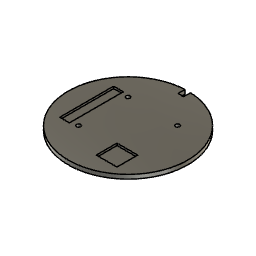
ASMBLY_NonSym v9 (Autodesk Fusion 360 archive; units mm, degrees)
design "Plate_Tag"
Autodesk Fusion 360 part; units mm, degrees
(part 1 of 2)
sketch "Sketch1" plane through (0, 0, 0) normal (0, 0, 1) x (1, 0, 0)
  circle A0 centre (0, 0) radius 43.3
  line L0 (17.936, 17.936) -> (-17.936, 17.936) construction
  line L1 (-17.936, 17.936) -> (-17.936, -17.936) construction
  line L2 (-17.936, -17.936) -> (17.936, -17.936) construction
  line L3 (17.936, -17.936) -> (17.936, 17.936) construction
  line L4 (17.936, 17.936) -> (-17.936, -17.936) construction
  line L5 (-17.936, 17.936) -> (17.936, -17.936) construction
  circle A1 centre (17.936, 17.936) radius 1.5
  line L6 (0, 17.936) -> (0, -17.936) construction
  line L7 (-17.936, 0) -> (17.936, 0) construction
  circle A2 centre (-17.936, 17.936) radius 1.5
  circle A3 centre (17.936, -17.936) radius 1.5
  circle A4 centre (-17.936, -17.936) radius 1.5
  line L8 (0, 43.3) -> (0, 38.2538) construction
  line L9 (0, 38.2538) -> (2, 38.2538)
  line L10 (2, 38.2538) -> (2, 43.2538)
  line L11 (-2, 38.2538) -> (-2, 43.2538)
  line L12 (0, 38.2538) -> (-2, 38.2538)
  line L13 (-23.936, 19.5) -> (-29.936, 19.5)
  line L14 (-29.936, 19.5) -> (-29.936, -19.5)
  line L15 (-29.936, -19.5) -> (-23.936, -19.5)
  line L16 (-23.936, -19.5) -> (-23.936, 19.5)
  line L17 (-23.936, 19.5) -> (-29.936, -19.5) construction
  line L18 (-29.936, 19.5) -> (-23.936, -19.5) construction
  point P0 (-26.936, 0)
  dimension "d1" = 86.6
  dimension "d2" = 35.872
  dimension "d3" = 35.872
  dimension "d4" = 3
  dimension "d7" = 4
  dimension "d8" = 5
  dimension "d9" = 6
  dimension "d10" = 39
  dimension "d26" = 12
  constraint coincident A0.centre origin
  constraint perpendicular L0 L1
  constraint parallel L0 L2
  constraint parallel L1 L3
  constraint horizontal L0
  constraint coincident L4 A0.centre
  constraint coincident L5 A0.centre
  constraint coincident L0.start L3.end
  constraint midpoint L0 L6.start
  constraint midpoint L2 L6.end
  constraint midpoint L1 L7.start
  constraint midpoint L3 L7.end
  constraint symmetric A1 L6 A2
  constraint symmetric A1 L7 A3
  constraint symmetric L7 A2 A4
  constraint coincident A0 L8.start
  constraint vertical L8
  constraint perpendicular L8 L9
  constraint coincident A0 L10.end
  constraint perpendicular L9 L10
  constraint collinear A0.centre L8.start L8.end
  constraint symmetric L9.start L8 L12.start
  constraint symmetric L8 L9.end L11.start
  constraint symmetric L8 L10.end L11.end
  constraint perpendicular L13 L14
  constraint parallel L13 L15
  constraint parallel L14 L16
  constraint horizontal L13
  constraint coincident L17 P0
  constraint coincident L18 P0
  constraint coincident L7 P0
  measures "d1" diameter of A0
  measures "d2" distance of L0.start L2.end
  measures "d3" distance of L0.start L0.end
  measures "d4" diameter of A1
  measures "d7" distance of L9.end L11.start
  measures "d8" distance of L9.end L10.end
  measures "d9" distance of L13.start L13.end
  measures "d10" distance of L13.end L14.end
  measures "d23" distance of A0.centre
  measures "d26" distance of L0.end L14
extrude "Extrude1" add sketch "Sketch1" along normal blind 3 contours A0 L9 L10 L11 L12 | A3 | L13 L14 L15 L16 picked at (5.5765, -5.6181)
sketch "Sketch2" plane through (0, 0, 3) normal (0, 0, 1) x (-1, 0, 0)
  circle A0 centre (17.936, 17.936) radius 1.5
  circle A1 centre (17.936, -17.936) radius 1.5
  circle A2 centre (-17.936, -17.936) radius 1.5
  line L0 (-2, -38.2538) -> (2, -38.2538)
  line L1 (2, -38.2538) -> (2, -43.2538)
  arc A3 (2, -43.2538) -> (-2, -43.2538) centre (0, 0) ccw
  line L2 (-2, -43.2538) -> (-2, -38.2538)
  line L3 (0, 0) -> (0, -19.5) construction
  line L4 (22.936, -19.5) -> (29.936, -19.5)
  line L5 (29.936, -19.5) -> (29.936, 19.5)
  line L6 (29.936, 19.5) -> (22.936, 19.5)
  line L7 (22.936, 19.5) -> (22.936, -19.5)
  line L8 (22.936, -19.5) -> (29.936, 19.5) construction
  line L9 (29.936, -19.5) -> (22.936, 19.5) construction
  line L10 (43.3, 0) -> (-43.3, 0) construction
  line L11 (-7, 15) -> (-22, 15)
  line L12 (-22, 15) -> (-22, 30)
  line L13 (-22, 30) -> (-7, 30)
  line L14 (-7, 30) -> (-7, 15)
  point P0 (26.436, 0)
  dimension "d12" = 7
  dimension "d13" = 39
  dimension "d22" = 15
  dimension "d23" = 15
  dimension "d24" = 15
  dimension "d25" = 7
  dimension "d27" = 12
  constraint coincident A3.centre L3.start
  constraint vertical L3
  constraint perpendicular L4 L5
  constraint parallel L4 L6
  constraint parallel L5 L7
  constraint horizontal L4
  constraint coincident L8 P0
  constraint coincident L9 P0
  constraint collinear L3.end L4.start L4.end
  constraint perpendicular L3 L10
  constraint midpoint A3.centre L10
  constraint coincident P0 L10
  constraint horizontal L11
  constraint vertical L12
  constraint horizontal L13
  constraint vertical L14
  constraint coincident A3 L10.end
  measures "d12" distance of L4.start L4.end
  measures "d13" distance of L4.end L5.end
  measures "d22" distance of L12.end L13.end A3.centre
  measures "d23" distance of L11.end L12.end A3.centre
  measures "d24" distance of L10 L11 A3.centre
  measures "d25" distance of A3.centre L14
  measures "d27" distance of A1.centre L5
extrude "Extrude2" cut sketch "Sketch2" against normal blind 1.5 contours L4 L5 L6 L7 | L11 L12 L13 L14

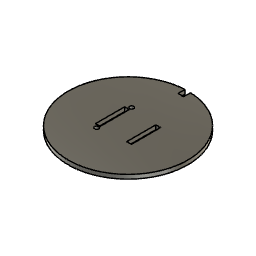
design "Plate_BNO"
Autodesk Fusion 360 part; units mm, degrees
sketch "Sketch1" plane through (0, 0, 0) normal (0, 0, 1) x (1, 0, 0)
  circle A0 centre (0, 0) radius 43.3
  line L0 (10, 12.7) -> (-10, 12.7) construction
  line L1 (-10, 12.7) -> (-10, -12.7) construction
  line L2 (-10, -12.7) -> (10, -12.7) construction
  line L3 (10, -12.7) -> (10, 12.7) construction
  line L4 (10, 12.7) -> (-10, -12.7) construction
  line L5 (-10, 12.7) -> (10, -12.7) construction
  line L6 (0, 12.7) -> (0, -12.7) construction
  line L7 (-10, 0) -> (10, 0) construction
  circle A1 centre (-10, 12.7) radius 1.5
  circle A2 centre (-10, -12.7) radius 1.5
  line L8 (-13, 10.5) -> (-9.6, 10.5)
  line L9 (-9.6, 10.5) -> (-9.6, -10.5)
  line L10 (-9.6, -10.5) -> (-13, -10.5)
  line L11 (-13, -10.5) -> (-13, 10.5)
  line L12 (-13, 10.5) -> (-9.6, -10.5) construction
  line L13 (-9.6, 10.5) -> (-13, -10.5) construction
  line L14 (13, 15.75) -> (-13, 15.75) construction
  line L15 (-13, 15.75) -> (-13, -15.75) construction
  line L16 (-13, -15.75) -> (13, -15.75) construction
  line L17 (13, -15.75) -> (13, 15.75) construction
  line L18 (13, 15.75) -> (-13, -15.75) construction
  line L19 (-13, 15.75) -> (13, -15.75) construction
  line L20 (-2, 43.2538) -> (-2, 38.2538)
  line L21 (-2, 38.2538) -> (2, 38.2538)
  line L22 (2, 38.2538) -> (2, 43.2538)
  line L23 (9.6, 10.5) -> (13, -10.5) construction
  line L24 (13, 10.5) -> (9.6, -10.5) construction
  line L25 (13, -10.5) -> (13, 10.5)
  line L26 (9.6, 10.5) -> (9.6, -10.5)
  line L27 (13, 10.5) -> (9.6, 10.5)
  line L28 (9.6, -10.5) -> (13, -10.5)
  point P0 (-11.3, 0)
  dimension "d1" = 86.6
  dimension "d2" = 25.4
  dimension "d3" = 20
  dimension "d5" = 3
  dimension "d9" = 26
  dimension "d10" = 31.5
  dimension "d11" = 21
  dimension "d12" = 3.4
  dimension "d13" = 9.6
  dimension "d30" = 4
  dimension "d31" = 5
  dimension "d32" = 2
  constraint coincident A0.centre origin
  constraint perpendicular L0 L1
  constraint parallel L0 L2
  constraint parallel L1 L3
  constraint horizontal L0
  constraint coincident L4 A0.centre
  constraint coincident L5 A0.centre
  constraint midpoint L0 L6.start
  constraint midpoint L2 L6.end
  constraint midpoint L1 L7.start
  constraint midpoint L3 L7.end
  constraint symmetric L7 A1 A2
  constraint coincident L0.end L1.start
  constraint perpendicular L8 L9
  constraint parallel L8 L10
  constraint parallel L9 L11
  constraint horizontal L8
  constraint coincident L12 P0
  constraint coincident L13 P0
  constraint perpendicular L14 L15
  constraint parallel L14 L16
  constraint parallel L15 L17
  constraint horizontal L14
  constraint coincident L18 A0.centre
  constraint coincident L19 A0.centre
  constraint collinear L7.start L7.end P0
  constraint coincident A0 L20.start
  constraint vertical L20
  constraint perpendicular L20 L21
  constraint coincident A0 L22.end
  constraint perpendicular L21 L22
  constraint symmetric L6 L8.start L24.start
  constraint symmetric L6 L8.end L23.start
  constraint symmetric L6 L9.end L24.end
  constraint symmetric L6 L10.end L23.end
  measures "d1" diameter of A0
  measures "d2" distance of L0.start L2.end
  measures "d3" distance of L0.start L0.end
  measures "d5" diameter of A1
  measures "d9" distance of L14.start L14.end
  measures "d10" distance of L14.end L15.end
  measures "d11" distance of L8.end L9.end
  measures "d12" distance of L8.start L8.end
  measures "d13" distance of L6 L9
  measures "d30" distance of L20.end L21.end
  measures "d31" distance of L21.end L22.end
  measures "d32" distance of L6 L22
extrude "Extrude1" add sketch "Sketch1" along normal blind 3 contours A0 L20 L21 L22 picked at (23.1, 0)

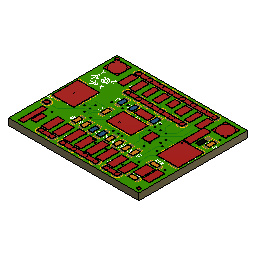
design "SparkFun_Qwiic_VR_IMU_Breakout"
part number: STAND-OFF
part number: FIDUCIALUFIDUCIAL
part number: SMD
part number: PTH
part number: 22pF
part number: OSHW-LOGOMINI
part number: BNO080
part number: 1k
part number: SPI
part number: 32.768kHz
part number: SFE_LOGO_FLAME.1_INCH
part number: SFE_LOGO_NAME_FLAME.1_INCH
part number: RED
Autodesk Fusion 360 part; units mm, degrees
sketch "sketch 305" plane through (0, 0, 0) normal (0, 0, 1) x (1, 0, 0)
  line L0 (0, 0) -> (0, 25.4)
  line L1 (0, 25.4) -> (30.48, 25.4)
  line L2 (30.48, 25.4) -> (30.48, 0)
  line L3 (30.48, 0) -> (0, 0)
extrude "Board" add sketch "sketch 305" along normal blind 1.57 makes body 1 in component "Board"
sketch "sketch 883" plane through (0, 0, 0) normal (0, 0, 1) x (1, 0, 0)
  line L0 (-1.651, -1.651) -> (1.651, -1.651)
  line L1 (1.651, -1.651) -> (1.651, 1.651)
  line L2 (1.651, 1.651) -> (-1.651, 1.651)
  line L3 (-1.651, 1.651) -> (-1.651, -1.651)
extrude "STAND-OFF" add sketch "sketch 883" along normal blind 0.1 separate body makes body 2 in component "STAND-OFF"
sketch "sketch 1039" plane through (0, 0, 0) normal (0, 0, 1) x (1, 0, 0)
  line L0 (-0.3175, -0.3175) -> (0.3175, -0.3175)
  line L1 (0.3175, -0.3175) -> (0.3175, 0.3175)
  line L2 (0.3175, 0.3175) -> (-0.3175, 0.3175)
  line L3 (-0.3175, 0.3175) -> (-0.3175, -0.3175)
extrude "MICRO-FIDUCIAL" add sketch "sketch 1039" along normal blind 0.1 separate body makes body 3 in component "MICRO-FIDUCIAL"
sketch "sketch 1179" plane through (0, 0, 0) normal (0, 0, 1) x (1, 0, 0)
  line L0 (-3, -4.6) -> (3, -4.6)
  line L1 (3, -4.6) -> (3, 0.441)
  line L2 (3, 0.441) -> (-3, 0.441)
  line L3 (-3, 0.441) -> (-3, -4.6)
extrude "1X04_1MM_RA" add sketch "sketch 1179" along normal blind 0.1 separate body makes body 4 in component "1X04_1MM_RA"
sketch "sketch 1311" plane through (0, 0, 0) normal (0, 0, 1) x (1, 0, 0)
  line L0 (-0.508, -0.508) -> (8.128, -0.508)
  line L1 (8.128, -0.508) -> (8.128, 0.508)
  line L2 (8.128, 0.508) -> (-0.508, 0.508)
  line L3 (-0.508, 0.508) -> (-0.508, -0.508)
extrude "1X04_NO_SILK" add sketch "sketch 1311" along normal blind 0.1 separate body makes body 5 in component "1X04_NO_SILK"
sketch "sketch 1475" plane through (0, 0, 0) normal (0, 0, 1) x (1, 0, 0)
  line L0 (-0.838, -0.47) -> (0.83, -0.47)
  line L1 (0.83, -0.47) -> (0.83, 0.48)
  line L2 (0.83, 0.48) -> (-0.838, 0.48)
  line L3 (-0.838, 0.48) -> (-0.838, -0.47)
extrude "0603" add sketch "sketch 1475" along normal blind 0.1 separate body makes body 6 in component "0603"
sketch "sketch 1607" plane through (0, 0, 0) normal (0, 0, 1) x (1, 0, 0)
  line L0 (-1.233, -0.993) -> (1.237, -0.993)
  line L1 (1.237, -0.993) -> (1.237, 1.217)
  line L2 (1.237, 1.217) -> (-1.233, 1.217)
  line L3 (-1.233, 1.217) -> (-1.233, -0.993)
extrude "OSHW-LOGO-MINI" add sketch "sketch 1607" along normal blind 0.1 separate body makes body 7 in component "OSHW-LOGO-MINI"
sketch "sketch 1739" plane through (0, 0, 0) normal (0, 0, 1) x (1, 0, 0)
  line L0 (-2, -2.7) -> (2, -2.7)
  line L1 (2, -2.7) -> (2, 3.101)
  line L2 (2, 3.101) -> (-2, 3.101)
  line L3 (-2, 3.101) -> (-2, -2.7)
extrude "LGA-28" add sketch "sketch 1739" along normal blind 0.1 separate body makes body 8 in component "LGA-28"
sketch "sketch 1943" plane through (0, 0, 0) normal (0, 0, 1) x (1, 0, 0)
  line L0 (-0.838, -0.47) -> (0.83, -0.47)
  line L1 (0.83, -0.47) -> (0.83, 0.48)
  line L2 (0.83, 0.48) -> (-0.838, 0.48)
  line L3 (-0.838, 0.48) -> (-0.838, -0.47)
extrude "0603'" add sketch "sketch 1943" along normal blind 0.1 separate body makes body 9 in component "0603 (1)"
sketch "sketch 2091" plane through (0, 0, 0) normal (0, 0, 1) x (1, 0, 0)
  line L0 (-1, -1) -> (1, -1)
  line L1 (1, -1) -> (1, 1)
  line L2 (1, 1) -> (-1, 1)
  line L3 (-1, 1) -> (-1, -1)
extrude "SJ_2S-NO" add sketch "sketch 2091" along normal blind 0.1 separate body makes body 10 in component "SJ_2S-NO"
sketch "sketch 2223" plane through (0, 0, 0) normal (0, 0, 1) x (1, 0, 0)
  line L0 (-1.524, -1.016) -> (1.524, -1.016)
  line L1 (1.524, -1.016) -> (1.524, 1.016)
  line L2 (1.524, 1.016) -> (-1.524, 1.016)
  line L3 (-1.524, 1.016) -> (-1.524, -1.016)
extrude "SMT-JUMPER_3_2-NC_PASTE_SILK" add sketch "sketch 2223" along normal blind 0.1 separate body makes body 11 in component "SMT-JUMPER_3_2-NC_PASTE_SILK"
sketch "sketch 2355" plane through (0, 0, 0) normal (0, 0, 1) x (1, 0, 0)
  line L0 (-0.508, -0.508) -> (18.288, -0.508)
  line L1 (18.288, -0.508) -> (18.288, 0.508)
  line L2 (18.288, 0.508) -> (-0.508, 0.508)
  line L3 (-0.508, 0.508) -> (-0.508, -0.508)
extrude "1X08_NO_SILK" add sketch "sketch 2355" along normal blind 0.1 separate body makes body 12 in component "1X08_NO_SILK"
sketch "sketch 2495" plane through (0, 0, 0) normal (0, 0, 1) x (1, 0, 0)
  line L0 (-0.508, -0.508) -> (3.048, -0.508)
  line L1 (3.048, -0.508) -> (3.048, 0.508)
  line L2 (3.048, 0.508) -> (-0.508, 0.508)
  line L3 (-0.508, 0.508) -> (-0.508, -0.508)
extrude "1X02_NO_SILK" add sketch "sketch 2495" along normal blind 0.1 separate body makes body 13 in component "1X02_NO_SILK"
sketch "sketch 2627" plane through (0, 0, 0) normal (0, 0, 1) x (1, 0, 0)
  line L0 (-0.508, -0.508) -> (13.208, -0.508)
  line L1 (13.208, -0.508) -> (13.208, 0.508)
  line L2 (13.208, 0.508) -> (-0.508, 0.508)
  line L3 (-0.508, 0.508) -> (-0.508, -0.508)
extrude "1X06_NO_SILK" add sketch "sketch 2627" along normal blind 0.1 separate body makes body 14 in component "1X06_NO_SILK"
sketch "sketch 2759" plane through (0, 0, 0) normal (0, 0, 1) x (1, 0, 0)
  line L0 (-0.508, -0.508) -> (0.508, -0.508)
  line L1 (0.508, -0.508) -> (0.508, 0.508)
  line L2 (0.508, 0.508) -> (-0.508, 0.508)
  line L3 (-0.508, 0.508) -> (-0.508, -0.508)
extrude "1X01_NO_SILK" add sketch "sketch 2759" along normal blind 0.1 separate body makes body 15 in component "1X01_NO_SILK"
sketch "sketch 2891" plane through (0, 0, 0) normal (0, 0, 1) x (1, 0, 0)
  line L0 (-1.6, -0.85) -> (1.6, -0.85)
  line L1 (1.6, -0.85) -> (1.6, 0.85)
  line L2 (1.6, 0.85) -> (-1.6, 0.85)
  line L3 (-1.6, 0.85) -> (-1.6, -0.85)
extrude "CRYSTAL-SMD-3.2X1.5MM" add sketch "sketch 2891" along normal blind 0.1 separate body makes body 16 in component "CRYSTAL-SMD-3.2X1.5MM"
sketch "sketch 3031" plane through (0, 0, 0) normal (0, 0, 1) x (1, 0, 0)
  line L0 (0.64, -0.82) -> (4.12, -0.82)
  line L1 (4.12, -0.82) -> (4.12, 0.82)
  line L2 (4.12, 0.82) -> (0.64, 0.82)
  line L3 (0.64, 0.82) -> (0.64, -0.82)
extrude "#RST>" add sketch "sketch 3031" along normal blind 0.1 separate body makes body 17 in component "#RST>"
sketch "sketch 3171" plane through (0, 0, 0) normal (0, 0, 1) x (1, 0, 0)
  line L0 (0.48, -0.82) -> (4.36, -0.82)
  line L1 (4.36, -0.82) -> (4.36, 0.82)
  line L2 (4.36, 0.82) -> (0.48, 0.82)
  line L3 (0.48, 0.82) -> (0.48, -0.82)
extrude "SCL" add sketch "sketch 3171" along normal blind 0.1 separate body makes body 18 in component "SCL"
sketch "sketch 3311" plane through (0, 0, 0) normal (0, 0, 1) x (1, 0, 0)
  line L0 (0.48, -0.82) -> (4.6, -0.82)
  line L1 (4.6, -0.82) -> (4.6, 0.82)
  line L2 (4.6, 0.82) -> (0.48, 0.82)
  line L3 (0.48, 0.82) -> (0.48, -0.82)
extrude "SDA" add sketch "sketch 3311" along normal blind 0.1 separate body makes body 19 in component "SDA"
sketch "sketch 3451" plane through (0, 0, 0) normal (0, 0, 1) x (1, 0, 0)
  line L0 (0.52, -0.82) -> (4.16, -0.82)
  line L1 (4.16, -0.82) -> (4.16, 0.82)
  line L2 (4.16, 0.82) -> (0.52, 0.82)
  line L3 (0.52, 0.82) -> (0.52, -0.82)
extrude "3V3" add sketch "sketch 3451" along normal blind 0.1 separate body makes body 20 in component "3V3"
sketch "sketch 3591" plane through (0, 0, 0) normal (0, 0, 1) x (1, 0, 0)
  line L0 (0.48, -0.82) -> (4.36, -0.82)
  line L1 (4.36, -0.82) -> (4.36, 0.82)
  line L2 (4.36, 0.82) -> (0.48, 0.82)
  line L3 (0.48, 0.82) -> (0.48, -0.82)
extrude "GND" add sketch "sketch 3591" along normal blind 0.1 separate body makes body 21 in component "GND"
sketch "sketch 3723" plane through (0, 0, 0) normal (0, 0, 1) x (1, 0, 0)
  line L0 (0.08, -0.82) -> (3.72, -0.82)
  line L1 (3.72, -0.82) -> (3.72, 0.82)
  line L2 (3.72, 0.82) -> (0.08, 0.82)
  line L3 (0.08, 0.82) -> (0.08, -0.82)
extrude "(I_SUPER2_C)" add sketch "sketch 3723" along normal blind 0.1 separate body makes body 22 in component "(I_SUPER2_C)"
sketch "sketch 3863" plane through (0, 0, 0) normal (0, 0, 1) x (1, 0, 0)
  line L0 (0.68, -0.82) -> (3.92, -0.82)
  line L1 (3.92, -0.82) -> (3.92, 0.82)
  line L2 (3.92, 0.82) -> (0.68, 0.82)
  line L3 (0.68, 0.82) -> (0.68, -0.82)
extrude "#INT0" add sketch "sketch 3863" along normal blind 0.1 separate body makes body 23 in component "#INT0"
sketch "sketch 4003" plane through (0, 0, 0) normal (0, 0, 1) x (1, 0, 0)
  line L0 (0.48, -0.82) -> (4.04, -0.82)
  line L1 (4.04, -0.82) -> (4.04, 0.82)
  line L2 (4.04, 0.82) -> (0.48, 0.82)
  line L3 (0.48, 0.82) -> (0.48, -0.82)
extrude "PS14" add sketch "sketch 4003" along normal blind 0.1 separate body makes body 24 in component "PS14"
sketch "sketch 4135" plane through (0, 0, 0) normal (0, 0, 1) x (1, 0, 0)
  line L0 (0.52, -0.82) -> (4.32, -0.82)
  line L1 (4.32, -0.82) -> (4.32, 0.82)
  line L2 (4.32, 0.82) -> (0.52, 0.82)
  line L3 (0.52, 0.82) -> (0.52, -0.82)
extrude "PS05" add sketch "sketch 4135" along normal blind 0.1 separate body makes body 25 in component "PS05"
sketch "sketch 4267" plane through (0, 0, 0) normal (0, 0, 1) x (1, 0, 0)
  line L0 (0.96, -0.58) -> (3.16, -0.58)
  line L1 (3.16, -0.58) -> (3.16, 0.54)
  line L2 (3.16, 0.54) -> (0.96, 0.54)
  line L3 (0.96, 0.54) -> (0.96, -0.58)
extrude "PS114" add sketch "sketch 4267" along normal blind 0.1 separate body makes body 26 in component "PS114"
sketch "sketch 4399" plane through (0, 0, 0) normal (0, 0, 1) x (1, 0, 0)
  line L0 (0.96, -0.58) -> (3.52, -0.58)
  line L1 (3.52, -0.58) -> (3.52, 0.54)
  line L2 (3.52, 0.54) -> (0.96, 0.54)
  line L3 (0.96, 0.54) -> (0.96, -0.58)
extrude "PS015" add sketch "sketch 4399" along normal blind 0.1 separate body makes body 27 in component "PS015"
sketch "sketch 4531" plane through (0, 0, 0) normal (0, 0, 1) x (1, 0, 0)
  line L0 (1.2, -0.73) -> (6.1, -0.73)
  line L1 (6.1, -0.73) -> (6.1, 0.68)
  line L2 (6.1, 0.68) -> (1.2, 0.68)
  line L3 (1.2, 0.68) -> (1.2, -0.73)
extrude "UART8" add sketch "sketch 4531" along normal blind 0.1 separate body makes body 28 in component "UART8"
sketch "sketch 4663" plane through (0, 0, 0) normal (0, 0, 1) x (1, 0, 0)
  line L0 (1.08, -0.58) -> (4, -0.58)
  line L1 (4, -0.58) -> (4, 0.54)
  line L2 (4, 0.54) -> (1.08, 0.54)
  line L3 (1.08, 0.54) -> (1.08, -0.58)
extrude "GRN10" add sketch "sketch 4663" along normal blind 0.1 separate body makes body 29 in component "GRN10"
sketch "sketch 4795" plane through (0, 0, 0) normal (0, 0, 1) x (1, 0, 0)
  line L0 (0.96, -0.54) -> (3.56, -0.54)
  line L1 (3.56, -0.54) -> (3.56, 0.54)
  line L2 (3.56, 0.54) -> (0.96, 0.54)
  line L3 (0.96, 0.54) -> (0.96, -0.54)
extrude "BLK9" add sketch "sketch 4795" along normal blind 0.1 separate body makes body 30 in component "BLK9"
sketch "sketch 4927" plane through (0, 0, 0) normal (0, 0, 1) x (1, 0, 0)
  line L0 (1.68, -1.02) -> (16.73, -1.02)
  line L1 (16.73, -1.02) -> (16.73, 0.95)
  line L2 (16.73, 0.95) -> (1.68, 0.95)
  line L3 (1.68, 0.95) -> (1.68, -1.02)
extrude "BNO080_IMU11" add sketch "sketch 4927" along normal blind 0.1 separate body makes body 31 in component "BNO080_IMU11"
sketch "sketch 5059" plane through (0, 0, 0) normal (0, 0, 1) x (1, 0, 0)
  line L0 (0.96, -0.58) -> (6.56, -0.58)
  line L1 (6.56, -0.58) -> (6.56, 0.54)
  line L2 (6.56, 0.54) -> (0.96, 0.54)
  line L3 (0.96, 0.54) -> (0.96, -0.58)
extrude "BNO08012" add sketch "sketch 5059" along normal blind 0.1 separate body makes body 32 in component "BNO08012"
sketch "sketch 5191" plane through (0, 0, 0) normal (0, 0, 1) x (1, 0, 0)
  line L0 (0.96, -0.58) -> (3.52, -0.58)
  line L1 (3.52, -0.58) -> (3.52, 0.54)
  line L2 (3.52, 0.54) -> (0.96, 0.54)
  line L3 (0.96, 0.54) -> (0.96, -0.58)
extrude "IMU13" add sketch "sketch 5191" along normal blind 0.1 separate body makes body 33 in component "IMU13"
sketch "sketch 5331" plane through (0, 0, 0) normal (0, 0, 1) x (1, 0, 0)
  line L0 (0.46, -0.72) -> (3.64, -0.72)
  line L1 (3.64, -0.72) -> (3.64, 0.72)
  line L2 (3.64, 0.72) -> (0.46, 0.72)
  line L3 (0.46, 0.72) -> (0.46, -0.72)
extrude "3V30" add sketch "sketch 5331" along normal blind 0.1 separate body makes body 34 in component "3V30"
sketch "sketch 5471" plane through (0, 0, 0) normal (0, 0, 1) x (1, 0, 0)
  line L0 (0.21, -0.72) -> (3.26, -0.72)
  line L1 (3.26, -0.72) -> (3.26, 0.72)
  line L2 (3.26, 0.72) -> (0.21, 0.72)
  line L3 (0.21, 0.72) -> (0.21, -0.72)
extrude "#RST7" add sketch "sketch 5471" along normal blind 0.1 separate body makes body 35 in component "#RST7"
sketch "sketch 5611" plane through (0, 0, 0) normal (0, 0, 1) x (1, 0, 0)
  line L0 (0.18, -0.61) -> (3.27, -0.61)
  line L1 (3.27, -0.61) -> (3.27, 0.61)
  line L2 (3.27, 0.61) -> (0.18, 0.61)
  line L3 (0.18, 0.61) -> (0.18, -0.61)
extrude "#WAK6" add sketch "sketch 5611" along normal blind 0.1 separate body makes body 36 in component "#WAK6"
sketch "sketch 5751" plane through (0, 0, 0) normal (0, 0, 1) x (1, 0, 0)
  line L0 (0.42, -0.72) -> (3.82, -0.72)
  line L1 (3.82, -0.72) -> (3.82, 0.72)
  line L2 (3.82, 0.72) -> (0.42, 0.72)
  line L3 (0.42, 0.72) -> (0.42, -0.72)
extrude "GND1" add sketch "sketch 5751" along normal blind 0.1 separate body makes body 37 in component "GND1"
sketch "sketch 5891" plane through (0, 0, 0) normal (0, 0, 1) x (1, 0, 0)
  line L0 (0.28, -0.82) -> (2.96, -0.82)
  line L1 (2.96, -0.82) -> (2.96, 0.82)
  line L2 (2.96, 0.82) -> (0.28, 0.82)
  line L3 (0.28, 0.82) -> (0.28, -0.82)
extrude "#CS3" add sketch "sketch 5891" along normal blind 0.1 separate body makes body 38 in component "#CS3"
sketch "sketch 6031" plane through (0, 0, 0) normal (0, 0, 1) x (1, 0, 0)
  line L0 (0.06, -0.61) -> (3.03, -0.61)
  line L1 (3.03, -0.61) -> (3.03, 0.61)
  line L2 (3.03, 0.61) -> (0.06, 0.61)
  line L3 (0.06, 0.61) -> (0.06, -0.61)
extrude "SCK0" add sketch "sketch 6031" along normal blind 0.1 separate body makes body 39 in component "SCK0"
sketch "sketch 6171" plane through (0, 0, 0) normal (0, 0, 1) x (1, 0, 0)
  line L0 (0.07, -0.72) -> (2.21, -0.72)
  line L1 (2.21, -0.72) -> (2.21, 0.72)
  line L2 (2.21, 0.72) -> (0.07, 0.72)
  line L3 (0.07, 0.72) -> (0.07, -0.72)
extrude "SI1" add sketch "sketch 6171" along normal blind 0.1 separate body makes body 40 in component "SI1"
sketch "sketch 6311" plane through (0, 0, 0) normal (0, 0, 1) x (1, 0, 0)
  line L0 (0.07, -0.72) -> (2.84, -0.72)
  line L1 (2.84, -0.72) -> (2.84, 0.72)
  line L2 (2.84, 0.72) -> (0.07, 0.72)
  line L3 (0.07, 0.72) -> (0.07, -0.72)
extrude "SO0" add sketch "sketch 6311" along normal blind 0.1 separate body makes body 41 in component "SO0"
sketch "sketch 6443" plane through (0, 0, 0) normal (0, 0, 1) x (1, 0, 0)
  line L0 (0.46, -0.72) -> (3.78, -0.72)
  line L1 (3.78, -0.72) -> (3.78, 0.72)
  line L2 (3.78, 0.72) -> (0.46, 0.72)
  line L3 (0.46, 0.72) -> (0.46, -0.72)
extrude "PS03" add sketch "sketch 6443" along normal blind 0.1 separate body makes body 42 in component "PS03"
sketch "sketch 6575" plane through (0, 0, 0) normal (0, 0, 1) x (1, 0, 0)
  line L0 (0.69, -0.44) -> (2.82, -0.44)
  line L1 (2.82, -0.44) -> (2.82, 0.41)
  line L2 (2.82, 0.41) -> (0.69, 0.41)
  line L3 (0.69, 0.41) -> (0.69, -0.44)
extrude "3V32" add sketch "sketch 6575" along normal blind 0.1 separate body makes body 43 in component "3V32"
sketch "sketch 6707" plane through (0, 0, 0) normal (0, 0, 1) x (1, 0, 0)
  line L0 (0.72, -0.41) -> (2.4, -0.41)
  line L1 (2.4, -0.41) -> (2.4, 0.41)
  line L2 (2.4, 0.41) -> (0.72, 0.41)
  line L3 (0.72, 0.41) -> (0.72, -0.41)
extrude "RXI1" add sketch "sketch 6707" along normal blind 0.1 separate body makes body 44 in component "RXI1"
sketch "sketch 6839" plane through (0, 0, 0) normal (0, 0, 1) x (1, 0, 0)
  line L0 (0.69, -0.44) -> (3.06, -0.44)
  line L1 (3.06, -0.44) -> (3.06, 0.41)
  line L2 (3.06, 0.41) -> (0.69, 0.41)
  line L3 (0.69, 0.41) -> (0.69, -0.44)
extrude "TXO0" add sketch "sketch 6839" along normal blind 0.1 separate body makes body 45 in component "TXO0"
sketch "sketch 6971" plane through (0, 0, 0) normal (0, 0, 1) x (1, 0, 0)
  line L0 (0.92, -0.54) -> (3.92, -0.54)
  line L1 (3.92, -0.54) -> (3.92, 0.54)
  line L2 (3.92, 0.54) -> (0.92, 0.54)
  line L3 (0.92, 0.54) -> (0.92, -0.54)
extrude "ADR0" add sketch "sketch 6971" along normal blind 0.1 separate body makes body 46 in component "ADR0"
sketch "sketch 7103" plane through (0, 0, 0) normal (0, 0, 1) x (1, 0, 0)
  line L0 (0.32, 0.36) -> (2.01, 0.36)
  line L1 (2.01, 0.36) -> (2.01, 2.89)
  line L2 (2.01, 2.89) -> (0.32, 2.89)
  line L3 (0.32, 2.89) -> (0.32, 0.36)
extrude "SFE_LOGO_FLAME_.1" add sketch "sketch 7103" along normal blind 0.1 separate body makes body 47 in component "SFE_LOGO_FLAME_.1"
sketch "sketch 7235" plane through (0, 0, 0) normal (0, 0, 1) x (1, 0, 0)
  line L0 (0.44, 0.1) -> (11.33, 0.1)
  line L1 (11.33, 0.1) -> (11.33, 5.19)
  line L2 (11.33, 5.19) -> (0.44, 5.19)
  line L3 (0.44, 5.19) -> (0.44, 0.1)
extrude "SFE_LOGO_NAME_FLAME_.1" add sketch "sketch 7235" along normal blind 0.1 separate body makes body 48 in component "SFE_LOGO_NAME_FLAME_.1"
sketch "sketch 7367" plane through (0, 0, 0) normal (0, 0, 1) x (1, 0, 0)
  line L0 (0.46, -0.72) -> (5.11, -0.72)
  line L1 (5.11, -0.72) -> (5.11, 0.72)
  line L2 (5.11, 0.72) -> (0.46, 0.72)
  line L3 (0.46, 0.72) -> (0.46, -0.72)
extrude "BOOT2" add sketch "sketch 7367" along normal blind 0.1 separate body makes body 49 in component "BOOT2"
sketch "sketch 7499" plane through (0, 0, 0) normal (0, 0, 1) x (1, 0, 0)
  line L0 (-0.159, -0.476) -> (1.588, -0.476)
  line L1 (1.588, -0.476) -> (1.588, 0.476)
  line L2 (1.588, 0.476) -> (-0.159, 0.476)
  line L3 (-0.159, 0.476) -> (-0.159, -0.476)
extrude "LED-0603" add sketch "sketch 7499" along normal blind 0.1 separate body makes body 50 in component "LED-0603"
sketch "sketch 7631" plane through (0, 0, 0) normal (0, 0, 1) x (1, 0, 0)
  line L0 (0.08, -0.82) -> (4.92, -0.82)
  line L1 (4.92, -0.82) -> (4.92, 0.82)
  line L2 (4.92, 0.82) -> (0.08, 0.82)
  line L3 (0.08, 0.82) -> (0.08, -0.82)
extrude "(PWR)" add sketch "sketch 7631" along normal blind 0.1 separate body makes body 51 in component "(PWR)"
sketch "sketch 7763" plane through (0, 0, 0) normal (0, 0, 1) x (1, 0, 0)
  line L0 (-1.38, -1.9) -> (1.49, -1.9)
  line L1 (1.49, -1.9) -> (1.49, 1.9)
  line L2 (1.49, 1.9) -> (-1.38, 1.9)
  line L3 (-1.38, 1.9) -> (-1.38, -1.9)
extrude "QWIIC#LABEL#FULL#M#PNG" add sketch "sketch 7763" along normal blind 0.1 separate body makes body 52 in component "QWIIC#LABEL#FULL#M#PNG"
sketch "sketch 409" plane through (0, 0, 0) normal (0, 0, 1) x (1, 0, 0)
  circle A0 centre (7.62, 11.43) radius 0.1525
  circle A1 centre (11.43, 16.51) radius 0.1905
  circle A2 centre (13.97, 12.065) radius 0.1905
  circle A3 centre (14.859, 9.652) radius 0.1905
  circle A4 centre (23.749, 12.192) radius 0.1525
  circle A5 centre (25.4, 15.24) radius 0.1525
  circle A6 centre (24.13, 10.668) radius 0.1525
  circle A7 centre (14.224, 5.588) radius 0.1525
  circle A8 centre (12.319, 5.588) radius 0.1525
  circle A9 centre (2.54, 12.7) radius 0.1525
  circle A10 centre (28.94, 7.7) radius 0.1525
  circle A11 centre (3.81, 6.35) radius 0.1525
  circle A12 centre (8.89, 15.24) radius 0.1525
  circle A13 centre (19.05, 15.24) radius 0.1525
  circle A14 centre (11.43, 15.24) radius 0.1525
  circle A15 centre (29.21, 20.32) radius 0.1525
  circle A16 centre (21.59, 10.16) radius 0.1525
  circle A17 centre (9.525, 9.652) radius 0.1525
  circle A18 centre (7.62, 10.16) radius 0.1525
  circle A19 centre (21.59, 15.24) radius 0.1525
  circle A20 centre (20.32, 15.24) radius 0.1525
  circle A21 centre (17.018, 9.525) radius 0.1525
  circle A22 centre (17.78, 5.08) radius 0.1525
  circle A23 centre (22.86, 13.97) radius 0.1525
  circle A24 centre (19.05, 13.97) radius 0.1525
  circle A25 centre (6.35, 11.43) radius 0.1525
  circle A26 centre (24.13, 6.35) radius 0.1525
  circle A27 centre (7.62, 12.7) radius 0.1525
  circle A28 centre (22.86, 12.7) radius 0.1525
  circle A29 centre (19.05, 16.51) radius 0.1525
  circle A30 centre (22.86, 3.81) radius 0.1525
  circle A31 centre (16.002, 9.652) radius 0.1525
  circle A32 centre (15.24, 5.08) radius 0.1525
  circle A33 centre (21.59, 11.43) radius 0.1525
  circle A34 centre (2.54, 22.86) radius 1.651
  circle A35 centre (27.94, 22.86) radius 1.651
  circle A36 centre (11.43, 1.27) radius 0.508
  circle A37 centre (13.97, 1.27) radius 0.508
  circle A38 centre (16.51, 1.27) radius 0.508
  circle A39 centre (19.05, 1.27) radius 0.508
  circle A40 centre (6.35, 24.13) radius 0.508
  circle A41 centre (8.89, 24.13) radius 0.508
  circle A42 centre (11.43, 24.13) radius 0.508
  circle A43 centre (13.97, 24.13) radius 0.508
  circle A44 centre (16.51, 24.13) radius 0.508
  circle A45 centre (19.05, 24.13) radius 0.508
  circle A46 centre (21.59, 24.13) radius 0.508
  circle A47 centre (24.13, 24.13) radius 0.508
  circle A48 centre (21.59, 1.27) radius 0.508
  circle A49 centre (24.13, 1.27) radius 0.508
  circle A50 centre (8.89, 1.27) radius 0.508
  circle A51 centre (6.35, 1.27) radius 0.508
  circle A52 centre (8.89, 19.05) radius 0.508
  circle A53 centre (11.43, 19.05) radius 0.508
  circle A54 centre (13.97, 19.05) radius 0.508
  circle A55 centre (16.51, 19.05) radius 0.508
  circle A56 centre (19.05, 19.05) radius 0.508
  circle A57 centre (21.59, 19.05) radius 0.508
  circle A58 centre (1.27, 7.62) radius 0.508
extrude "Extrude2" cut sketch "sketch 409" along normal blind 1.57 bodies 1 in component "Board"
component "PCB Component" placed x (1, 0, 0) y (0, 1, 0) z (0, 0, 1) at (0, 0, 0)
component "Board" placed x (1, 0, 0) y (0, 1, 0) z (0, 0, 1) at (0, 0, 0) in component "PCB Component"
component "STAND-OFF" placed x (1, 0, 0) y (0, 1, 0) z (0, 0, 1) at (2.54, 22.86, 1.57) in component "PCB Component"
component "STAND-OFF" placed x (1, 0, 0) y (0, 1, 0) z (0, 0, 1) at (27.94, 22.86, 1.57) in component "PCB Component"
component "MICRO-FIDUCIAL" placed x (1, 0, 0) y (0, 1, 0) z (0, 0, 1) at (29.591, 0.889, 1.57) in component "PCB Component"
component "MICRO-FIDUCIAL" placed x (1, 0, 0) y (0, 1, 0) z (0, 0, 1) at (0.762, 24.638, 1.57) in component "PCB Component"
component "MICRO-FIDUCIAL" placed x (-1, 0, 0) y (0, 1, 0) z (0, 0, -1) at (29.591, 0.889, 0) in component "PCB Component"
component "MICRO-FIDUCIAL" placed x (-1, 0, 0) y (0, 1, 0) z (0, 0, -1) at (0.762, 24.638, 0) in component "PCB Component"
component "1X04_1MM_RA" placed x (0, -1, 0) y (1, 0, 0) z (0, 0, 1) at (5.08, 12.7, 1.57) in component "PCB Component"
component "1X04_1MM_RA" placed x (0, 1, 0) y (-1, 0, 0) z (0, 0, 1) at (25.4, 12.7, 1.57) in component "PCB Component"
component "1X04_NO_SILK" placed x (1, 0, 0) y (0, 1, 0) z (0, 0, 1) at (11.43, 1.27, 1.57) in component "PCB Component"
component "0603" placed x (0, -1, 0) y (1, 0, 0) z (0, 0, 1) at (14.224, 7.62, 1.57) in component "PCB Component"
component "0603" placed x (0, -1, 0) y (1, 0, 0) z (0, 0, 1) at (12.319, 7.62, 1.57) in component "PCB Component"
component "0603" placed x (0, 1, 0) y (-1, 0, 0) z (0, 0, 1) at (10.16, 16.51, 1.57) in component "PCB Component"
component "0603" placed x (0, -1, 0) y (1, 0, 0) z (0, 0, 1) at (17.78, 16.51, 1.57) in component "PCB Component"
component "0603" placed x (0, 1, 0) y (-1, 0, 0) z (0, 0, 1) at (12.7, 16.51, 1.57) in component "PCB Component"
component "OSHW-LOGO-MINI" placed x (-1, 0, 0) y (0, 1, 0) z (0, 0, -1) at (27.94, 2.54, 0) in component "PCB Component"
component "LGA-28" placed x (0, 1, 0) y (-1, 0, 0) z (0, 0, 1) at (15.24, 12.7, 1.57) in component "PCB Component"
component "0603 (1)" placed x (0, -1, 0) y (1, 0, 0) z (0, 0, 1) at (16.129, 7.62, 1.57) in component "PCB Component"
component "0603 (1)" placed x (0, -1, 0) y (1, 0, 0) z (0, 0, 1) at (21.844, 7.62, 1.57) in component "PCB Component"
component "0603 (1)" placed x (0, 1, 0) y (-1, 0, 0) z (0, 0, 1) at (10.16, 12.7, 1.57) in component "PCB Component"
component "0603 (1)" placed x (0, 1, 0) y (-1, 0, 0) z (0, 0, 1) at (10.414, 7.62, 1.57) in component "PCB Component"
component "0603 (1)" placed x (0, 1, 0) y (-1, 0, 0) z (0, 0, 1) at (8.509, 7.62, 1.57) in component "PCB Component"
component "0603 (1)" placed x (0, -1, 0) y (1, 0, 0) z (0, 0, 1) at (19.939, 7.62, 1.57) in component "PCB Component"
component "0603 (1)" placed x (0, -1, 0) y (1, 0, 0) z (0, 0, 1) at (18.034, 7.62, 1.57) in component "PCB Component"
component "0603 (1)" placed x (1, 0, 0) y (0, 1, 0) z (0, 0, 1) at (26.67, 7.62, 1.57) in component "PCB Component"
component "0603 (1)" placed x (1, 0, 0) y (0, 1, 0) z (0, 0, 1) at (26.67, 2.54, 1.57) in component "PCB Component"
component "0603 (1)" placed x (0, -1, 0) y (1, 0, 0) z (0, 0, 1) at (29.083, 18.288, 1.57) in component "PCB Component"
component "SJ_2S-NO" placed x (-1, 0, 0) y (0, 1, 0) z (0, 0, -1) at (24.13, 8.89, 0) in component "PCB Component"
component "SJ_2S-NO" placed x (1, 0, 0) y (0, -1, 0) z (0, 0, -1) at (6.35, 6.35, 0) in component "PCB Component"
component "SJ_2S-NO" placed x (1, 0, 0) y (0, -1, 0) z (0, 0, -1) at (6.35, 8.89, 0) in component "PCB Component"
component "SMT-JUMPER_3_2-NC_PASTE_SILK" placed x (0, -1, 0) y (1, 0, 0) z (0, 0, 1) at (26.67, 5.08, 1.57) in component "PCB Component"
component "1X08_NO_SILK" placed x (1, 0, 0) y (0, 1, 0) z (0, 0, 1) at (6.35, 24.13, 1.57) in component "PCB Component"
component "1X02_NO_SILK" placed x (1, 0, 0) y (0, 1, 0) z (0, 0, 1) at (21.59, 1.27, 1.57) in component "PCB Component"
component "1X02_NO_SILK" placed x (-1, 0, 0) y (0, -1, 0) z (0, 0, 1) at (8.89, 1.27, 1.57) in component "PCB Component"
component "1X06_NO_SILK" placed x (1, 0, 0) y (0, 1, 0) z (0, 0, 1) at (8.89, 19.05, 1.57) in component "PCB Component"
component "1X01_NO_SILK" placed x (1, 0, 0) y (0, 1, 0) z (0, 0, 1) at (1.27, 7.62, 1.57) in component "PCB Component"
component "CRYSTAL-SMD-3.2X1.5MM" placed x (-1, 0, 0) y (0, -1, 0) z (0, 0, 1) at (15.24, 16.51, 1.57) in component "PCB Component"
component "#RST>" placed x (0, 1, 0) y (-1, 0, 0) z (0, 0, 1) at (21.59, 1.524, 1.57) in component "PCB Component"
component "#RST>" placed x (0, 1, 0) y (1, 0, 0) z (0, 0, -1) at (21.59, 1.524, 0) in component "PCB Component"
component "SCL" placed x (0, 1, 0) y (1, 0, 0) z (0, 0, -1) at (19.05, 1.651, 0) in component "PCB Component"
component "SCL" placed x (0, 1, 0) y (-1, 0, 0) z (0, 0, 1) at (19.05, 1.651, 1.57) in component "PCB Component"
component "SDA" placed x (0, 1, 0) y (-1, 0, 0) z (0, 0, 1) at (16.51, 1.651, 1.57) in component "PCB Component"
component "SDA" placed x (0, 1, 0) y (1, 0, 0) z (0, 0, -1) at (16.51, 1.651, 0) in component "PCB Component"
component "3V3" placed x (0, 1, 0) y (1, 0, 0) z (0, 0, -1) at (13.97, 1.651, 0) in component "PCB Component"
component "3V3" placed x (0, 1, 0) y (-1, 0, 0) z (0, 0, 1) at (13.97, 1.651, 1.57) in component "PCB Component"
component "GND" placed x (0, 1, 0) y (-1, 0, 0) z (0, 0, 1) at (11.43, 1.651, 1.57) in component "PCB Component"
component "GND" placed x (0, 1, 0) y (1, 0, 0) z (0, 0, -1) at (11.43, 1.651, 0) in component "PCB Component"
component "(I_SUPER2_C)" placed x (0, 1, 0) y (-1, 0, 0) z (0, 0, 1) at (28.829, 3.175, 1.57) in component "PCB Component"
component "#INT0" placed x (0, 1, 0) y (-1, 0, 0) z (0, 0, 1) at (24.13, 1.524, 1.57) in component "PCB Component"
component "#INT0" placed x (0, 1, 0) y (1, 0, 0) z (0, 0, -1) at (24.13, 1.524, 0) in component "PCB Component"
component "PS14" placed x (0, 1, 0) y (1, 0, 0) z (0, 0, -1) at (8.89, 1.651, 0) in component "PCB Component"
component "PS14" placed x (0, 1, 0) y (-1, 0, 0) z (0, 0, 1) at (8.89, 1.651, 1.57) in component "PCB Component"
component "PS05" placed x (0, 1, 0) y (-1, 0, 0) z (0, 0, 1) at (6.35, 1.651, 1.57) in component "PCB Component"
component "PS114" placed x (0, 1, 0) y (1, 0, 0) z (0, 0, -1) at (4.064, 6.858, 0) in component "PCB Component"
component "PS015" placed x (0, 1, 0) y (1, 0, 0) z (0, 0, -1) at (4.064, 3.937, 0) in component "PCB Component"
component "UART8" placed x (-1, 0, 0) y (0, 1, 0) z (0, 0, -1) at (29.464, 18.034, 0) in component "PCB Component"
component "GRN10" placed x (-1, 0, 0) y (0, 1, 0) z (0, 0, -1) at (24.13, 17.018, 0) in component "PCB Component"
component "BLK9" placed x (-1, 0, 0) y (0, 1, 0) z (0, 0, -1) at (11.176, 17.018, 0) in component "PCB Component"
component "BNO080_IMU11" placed x (-1, 0, 0) y (0, 1, 0) z (0, 0, -1) at (24.511, 13.462, 0) in component "PCB Component"
component "BNO08012" placed x (0, 1, 0) y (-1, 0, 0) z (0, 0, 1) at (2.159, -0.254, 1.57) in component "PCB Component"
component "IMU13" placed x (0, 1, 0) y (-1, 0, 0) z (0, 0, 1) at (3.556, 1.27, 1.57) in component "PCB Component"
component "3V30" placed x (0, 1, 0) y (-1, 0, 0) z (0, 0, 1) at (8.89, 19.558, 1.57) in component "PCB Component"
component "3V30" placed x (0, 1, 0) y (1, 0, 0) z (0, 0, -1) at (8.89, 19.558, 0) in component "PCB Component"
component "#RST7" placed x (0, 1, 0) y (1, 0, 0) z (0, 0, -1) at (24.13, 19.939, 0) in component "PCB Component"
component "#RST7" placed x (0, 1, 0) y (-1, 0, 0) z (0, 0, 1) at (24.13, 19.939, 1.57) in component "PCB Component"
component "#WAK6" placed x (0, 1, 0) y (-1, 0, 0) z (0, 0, 1) at (21.59, 19.939, 1.57) in component "PCB Component"
component "#WAK6" placed x (0, 1, 0) y (1, 0, 0) z (0, 0, -1) at (21.59, 19.939, 0) in component "PCB Component"
component "GND1" placed x (0, 1, 0) y (1, 0, 0) z (0, 0, -1) at (6.35, 19.431, 0) in component "PCB Component"
component "GND1" placed x (0, 1, 0) y (-1, 0, 0) z (0, 0, 1) at (6.35, 19.431, 1.57) in component "PCB Component"
component "#CS3" placed x (0, 1, 0) y (-1, 0, 0) z (0, 0, 1) at (19.05, 20.193, 1.57) in component "PCB Component"
component "#CS3" placed x (0, 1, 0) y (1, 0, 0) z (0, 0, -1) at (19.05, 20.193, 0) in component "PCB Component"
component "SCK0" placed x (0, 1, 0) y (-1, 0, 0) z (0, 0, 1) at (11.43, 20.193, 1.57) in component "PCB Component"
component "SCK0" placed x (0, 1, 0) y (1, 0, 0) z (0, 0, -1) at (11.43, 20.193, 0) in component "PCB Component"
component "SI1" placed x (0, 1, 0) y (-1, 0, 0) z (0, 0, 1) at (16.51, 20.955, 1.57) in component "PCB Component"
component "SI1" placed x (0, 1, 0) y (1, 0, 0) z (0, 0, -1) at (16.51, 20.955, 0) in component "PCB Component"
component "SO0" placed x (0, 1, 0) y (1, 0, 0) z (0, 0, -1) at (13.97, 20.32, 0) in component "PCB Component"
component "SO0" placed x (0, 1, 0) y (-1, 0, 0) z (0, 0, 1) at (13.97, 20.32, 1.57) in component "PCB Component"
component "PS03" placed x (0, 1, 0) y (1, 0, 0) z (0, 0, -1) at (6.35, 1.651, 0) in component "PCB Component"
component "3V32" placed x (0, 1, 0) y (1, 0, 0) z (0, 0, -1) at (13.97, 14.732, 0) in component "PCB Component"
component "RXI1" placed x (0, 1, 0) y (1, 0, 0) z (0, 0, -1) at (16.51, 15.113, 0) in component "PCB Component"
component "TXO0" placed x (0, 1, 0) y (1, 0, 0) z (0, 0, -1) at (19.05, 14.478, 0) in component "PCB Component"
component "ADR0" placed x (0, 1, 0) y (1, 0, 0) z (0, 0, -1) at (26.289, 6.35, 0) in component "PCB Component"
component "SFE_LOGO_FLAME_.1" placed x (1, 0, 0) y (0, 1, 0) z (0, 0, 1) at (19.431, 11.049, 1.57) in component "PCB Component"
component "SFE_LOGO_NAME_FLAME_.1" placed x (-1, 0, 0) y (0, 1, 0) z (0, 0, -1) at (21.209, 6.35, 0) in component "PCB Component"
component "BOOT2" placed x (0, 1, 0) y (1, 0, 0) z (0, 0, -1) at (1.27, 8.128, 0) in component "PCB Component"
component "LED-0603" placed x (0, -1, 0) y (1, 0, 0) z (0, 0, 1) at (27.559, 18.288, 1.57) in component "PCB Component"
component "(PWR)" placed x (0, 1, 0) y (-1, 0, 0) z (0, 0, 1) at (25.781, 15.875, 1.57) in component "PCB Component"
component "QWIIC#LABEL#FULL#M#PNG" placed x (-1, 0, 0) y (0, 1, 0) z (0, 0, -1) at (27.305, 13.208, 0) in component "PCB Component"
named bodies: "Board", "STAND-OFF", "MICRO-FIDUCIAL", "1X04_1MM_RA", "1X04_NO_SILK", "0603", "OSHW-LOGO-MINI", "LGA-28", "SJ_2S-NO", "SMT-JUMPER_3_2-NC_PASTE_SILK", "1X08_NO_SILK", "1X02_NO_SILK", "1X06_NO_SILK", "1X01_NO_SILK", "CRYSTAL-SMD-3.2X1.5MM", "#RST>", "SCL", "SDA", "3V3", "GND", "(I_SUPER2_C)", "#INT0", "PS14", "PS05", "PS114", "PS015", "UART8", "GRN10", "BLK9", "BNO080_IMU11", "BNO08012", "IMU13", "3V30", "#RST7", "#WAK6", "GND1", "#CS3", "SCK0", "SI1", "SO0", "PS03", "3V32", "RXI1", "TXO0", "ADR0", "SFE_LOGO_FLAME_.1", "SFE_LOGO_NAME_FLAME_.1", "BOOT2", "LED-0603", "(PWR)", "QWIIC#LABEL#FULL#M#PNG"

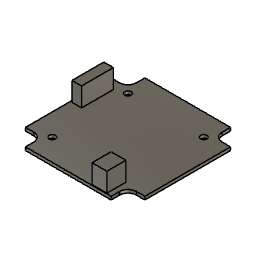
design "Pozyx_Tag"
Autodesk Fusion 360 part; units mm, degrees
sketch "Sketch1" plane through (0, 0, 0) normal (0, 0, 1) x (1, 0, 0)
  line L0 (0, 0) -> (0, 28.3) construction
  line L1 (0, 28.3) -> (20.3, 28.3)
  line L2 (28.3, 20.3) -> (28.3, 0)
  line L3 (0, 0) -> (28.3, 0) construction
  line L4 (28.3, 20.3) -> (24.3, 20.3)
  circle A0 centre (17.936, 17.936) radius 1.5
  line L5 (0, 28.3) -> (-20.3, 28.3)
  line L6 (-28.3, 20.3) -> (-24.3, 20.3)
  line L7 (-28.3, 20.3) -> (-28.3, 0)
  circle A1 centre (-17.936, 17.936) radius 1.5
  line L8 (0, -28.3) -> (-20.3, -28.3)
  line L9 (0, 0) -> (0, -28.3) construction
  line L10 (28.3, -20.3) -> (28.3, 0)
  line L11 (28.3, -20.3) -> (24.3, -20.3)
  line L12 (0, -28.3) -> (20.3, -28.3)
  circle A2 centre (-17.936, -17.936) radius 1.5
  line L13 (-28.3, -20.3) -> (-28.3, 0)
  line L14 (-28.3, -20.3) -> (-24.3, -20.3)
  circle A3 centre (17.936, -17.936) radius 1.5
  line L15 (20.3, 28.3) -> (20.3, 24.3)
  arc A4 (20.3, 24.3) -> (24.3, 20.3) centre (24.3, 24.3) ccw
  line L16 (24.3, 24.3) -> (17.936, 17.936) construction
  arc A5 (-24.3, 20.3) -> (-20.3, 24.3) centre (-24.3, 24.3) ccw
  line L17 (-20.3, 28.3) -> (-20.3, 24.3)
  line L18 (-20.3, -28.3) -> (-20.3, -24.3)
  arc A6 (-20.3, -24.3) -> (-24.3, -20.3) centre (-24.3, -24.3) ccw
  line L19 (20.3, -28.3) -> (20.3, -24.3)
  arc A7 (24.3, -20.3) -> (20.3, -24.3) centre (24.3, -24.3) ccw
  dimension "d3" = 28.3
  dimension "d4" = 28.3
  dimension "d6" = 8
  dimension "d7" = 8
  dimension "d8" = 4
  dimension "d9" = 3
  dimension "d15" = 4
  dimension "d16" = 45
  dimension "d17" = 9
  constraint coincident L0.start L3.start
  constraint vertical L0
  constraint coincident L0 L1.start
  constraint perpendicular L0 L1
  constraint perpendicular L1 L2
  constraint perpendicular L0 L3
  constraint coincident L2.end L3
  constraint perpendicular L2 L4
  constraint symmetric L0 L1.start L5.start
  constraint symmetric L0 L2.start L6.start
  constraint symmetric L0 L2.end L7.end
  constraint symmetric L0 L1.end L5.end
  constraint symmetric L0 L4.end L6.end
  constraint symmetric L0 A0 A1
  constraint symmetric L0.start L3 L9.start
  constraint symmetric L0.end L3 L8.start
  constraint symmetric L2.start L3 L10.start
  constraint symmetric L2.end L3 L10.end
  constraint symmetric L3 L1.end L12.end
  constraint symmetric L3 L4.end L11.end
  constraint symmetric L3 A0 A3
  constraint symmetric L3 L0.end L8.start
  constraint symmetric L3 L5.end L8.end
  constraint symmetric L3 L6.end L14.end
  constraint symmetric L3 L6.start L13.start
  constraint symmetric L3 L7.end L13.end
  constraint symmetric L3 A1 A2
  constraint perpendicular L1 L15
  constraint tangent L15 A4
  constraint coincident A4.centre L16.start
  constraint coincident A0.centre L16.end
  constraint symmetric L0 L15.end A5.end
  constraint symmetric L0 A4 A5
  constraint symmetric L3 L15.end L19.end
  constraint symmetric L3 A4 A7
  constraint symmetric L3 A5.end L18.end
  constraint symmetric L3 A5 A6
  constraint coincident L2.end L3.end
  constraint coincident L8.start L9.end
  measures "d3" distance of L0.start L1
  measures "d4" distance of L0.start L2
  measures "d6" distance of L2 L1.end
  measures "d7" distance of L2.start L1
  measures "d8" distance of L2.start L4.end
  measures "d9" diameter of A0
  measures "d15" distance of L1.end L15.end
  measures "d16" angle of L1 L16
  measures "d17" distance of A4.centre A0.centre
extrude "Extrude1" add sketch "Sketch1" along normal blind 1.5 contours L1 L2 L4 L5 L6 L7 L8 L10 L11 L12 L13 L14 L15 A4 A5 L17 L18 A6 L19 A7 | A3
sketch "Sketch2" plane through (0, 0, 1.5) normal (0, 0, 1) x (-1, 0, 0)
  circle A0 centre (17.936, 17.936) radius 1.5
  circle A1 centre (-17.936, -17.936) radius 1.5
  circle A2 centre (17.936, -17.936) radius 1.5
  line L0 (-28.3, 20.3) -> (-28.3, -20.3)
  line L1 (-28.3, -20.3) -> (-24.3, -20.3)
  arc A3 (-20.3, -24.3) -> (-24.3, -20.3) centre (-24.3, -24.3) ccw
  line L2 (-20.3, -24.3) -> (-20.3, -28.3)
  line L3 (-20.3, -28.3) -> (20.3, -28.3)
  line L4 (20.3, -28.3) -> (20.3, -24.3)
  arc A4 (24.3, -20.3) -> (20.3, -24.3) centre (24.3, -24.3) ccw
  line L5 (24.3, -20.3) -> (28.3, -20.3)
  line L6 (28.3, -20.3) -> (28.3, 20.3)
  line L7 (28.3, 20.3) -> (24.3, 20.3)
  arc A5 (20.3, 24.3) -> (24.3, 20.3) centre (24.3, 24.3) ccw
  line L8 (20.3, 24.3) -> (20.3, 28.3)
  line L9 (20.3, 28.3) -> (-20.3, 28.3)
  line L10 (-20.3, 28.3) -> (-20.3, 24.3)
  arc A6 (-24.3, 20.3) -> (-20.3, 24.3) centre (-24.3, 24.3) ccw
  line L11 (-24.3, 20.3) -> (-28.3, 20.3)
  line L12 (27.5365, -16.0729) -> (23, -16.0729)
  line L13 (23, -16.0729) -> (23, -1)
  line L14 (23, -1) -> (27.5365, -1)
  line L15 (27.5365, -1) -> (27.5365, -16.0729)
  line L16 (-11, 19) -> (-18, 19)
  line L17 (-18, 19) -> (-18, 28)
  line L18 (-18, 28) -> (-11, 28)
  line L19 (-11, 28) -> (-11, 19)
  constraint horizontal L12
  constraint vertical L13
  constraint horizontal L14
  constraint vertical L15
  constraint horizontal L16
  constraint vertical L17
  constraint horizontal L18
  constraint vertical L19
extrude "Extrude2" add sketch "Sketch2" along normal blind 9 contours L12 L13 L14 L15 | L16 L17 L18 L19

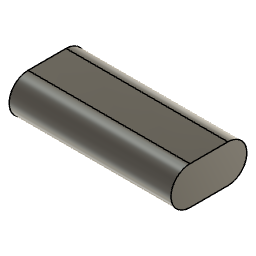
design "Battery"
Autodesk Fusion 360 part; units mm, degrees
sketch "Sketch1" plane through (0, 0, 0) normal (1, 0, 0) x (0, 1, 0)
  line L0 (11.25, 11.25) -> (-11.25, 11.25)
  line L1 (-11.25, -11.25) -> (11.25, -11.25)
  line L2 (22.5, 11.25) -> (-22.5, -11.25) construction
  line L3 (-22.5, 11.25) -> (22.5, -11.25) construction
  arc A0 (11.25, -11.25) -> (11.25, 11.25) centre (11.25, 0) ccw
  arc A1 (-11.25, 11.25) -> (-11.25, -11.25) centre (-11.25, 0) ccw
  line L4 (-22.5, 11.25) -> (-22.5, -11.25) construction
  line L5 (22.5, 11.25) -> (22.5, -11.25) construction
  line L6 (-22.5, 11.25) -> (22.5, 11.25) construction
  line L7 (-22.5, -11.25) -> (22.5, -11.25) construction
  dimension "d3" = 45
  dimension "d4" = 22.5
  constraint parallel L0 L1
  constraint horizontal L0
  constraint coincident L2 origin
  constraint coincident L3 origin
  constraint vertical L4
  constraint vertical L5
  constraint tangent L0 A0
  constraint tangent L0 A1
  constraint tangent L1 A1
  constraint tangent L1 A0
  constraint tangent A1 L4
  constraint tangent A0 L5
  constraint collinear L0 L6
  constraint collinear L1 L7
  measures "d3" distance of L4 L5
  measures "d4" distance of L2.start L3.end
extrude "Extrude1" add sketch "Sketch1" along normal blind 96

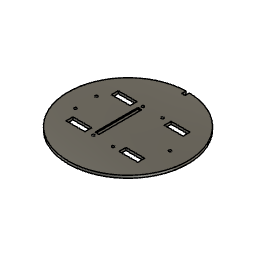
design "Plate_mid"
Autodesk Fusion 360 part; units mm, degrees